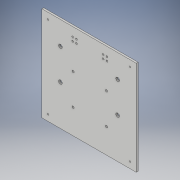
# Autodesk Inventor part: base_plate_v1
Saved by Autodesk Inventor 2019 (Build 230136000, 136)
## iProperties
Created: 2018-09-28
Part Number: base_plate_v1
Material: Generic
Document SubType Name: Modeling
Designer: Brian
Density: 1 g/cm^3
Appearance: Default
Author: Brian
Autodesk Inventor part; units mm, degrees
ref_plane "YZ Plane" through (0, 0, 0) normal (1, 0, 0) x (0, 1, 0)
ref_plane "XZ Plane" through (0, 0, 0) normal (0, 1, 0) x (-1, 0, 0)
ref_plane "XY Plane" through (0, 0, 0) normal (0, 0, 1) x (1, 0, 0)
sketch "Sketch1" plane through (0, 0, 0) normal (0, 0, 1) x (1, 0, 0)
  line L0 (0, 0) -> (304.8, 0)
  line L1 (304.8, 0) -> (304.8, 304.8)
  line L2 (304.8, 304.8) -> (0, 304.8)
  line L3 (0, 304.8) -> (0, 0)
  dimension "d0" = 304.8
  dimension "d1" = 304.8
  constraints: 8 end point, 2 parallel, 1 horizontal, 1 perpendicular
  measures "d0" distance of L2.end L1.end
  measures "d1" distance of L1.end L0.end
extrude "Extrusion1" add sketch "Sketch1" along normal blind 6
sketch "Sketch2" plane through (0, 0, 6) normal (0, 0, 1) x (1, 0, 0)
  line L0 (304.8, 0) -> (304.8, 304.8) projected
  line L1 (304.8, 304.8) -> (0, 304.8) projected
  point P0 (0, 0)
  point P1 (284.8, 284.8)
  dimension "d32" = 20
  dimension "d33" = 20
  measures "d32" distance from line of L0 point (284.8, 284.8)
  measures "d33" distance from line of L1 point (284.8, 284.8)
hole "Hole1" at (284.8, 284.8, 6) direction (0, 0, -1) diameter 5 end through all
sketch "Sketch3" plane through (0, 0, 6) normal (0, 0, 1) x (1, 0, 0)
  line L0 (0, 304.8) -> (0, 0) projected
  line L1 (304.8, 304.8) -> (0, 304.8) projected
  point P0 (20, 284.8)
  dimension "d34" = 20
  dimension "d35" = 20
  measures "d34" distance from line of L0 point (20, 284.8)
  measures "d35" distance from line of L1 point (20, 284.8)
hole "Hole2" at (20, 284.8, 6) direction (0, 0, -1) diameter 5 end through all
sketch "Sketch4" plane through (0, 0, 6) normal (0, 0, 1) x (1, 0, 0)
  line L0 (0, 0) -> (304.8, 0) projected
  line L1 (0, 304.8) -> (0, 0) projected
  point P0 (20, 20)
  dimension "d36" = 20
  dimension "d37" = 20
  measures "d36" distance from line of L0 point (20, 20)
  measures "d37" distance from line of L1 point (20, 20)
hole "Hole3" at (20, 20, 6) direction (0, 0, -1) diameter 5 end through all
sketch "Sketch5" plane through (0, 0, 6) normal (0, 0, 1) x (1, 0, 0)
  line L0 (0, 0) -> (304.8, 0) projected
  line L1 (304.8, 0) -> (304.8, 304.8) projected
  point P0 (284.8, 20)
  dimension "d38" = 20
  dimension "d39" = 20
  measures "d38" distance from line of L0 point (284.8, 20)
  measures "d39" distance from line of L1 point (284.8, 20)
hole "Hole4" at (284.8, 20, 6) direction (0, 0, -1) diameter 5 end through all
sketch "Sketch6" plane through (0, 0, 6) normal (0, 0, 1) x (1, 0, 0)
  line L0 (304.8, 304.8) -> (0, 304.8) projected
  line L1 (304.8, 0) -> (304.8, 304.8) projected
  point P0 (0, 0)
  point P1 (244.8, 229.8)
  dimension "d68" = 75
  dimension "d69" = 60
  measures "d68" distance from line of L0 point (244.8, 229.8)
  measures "d69" distance from line of L1 point (244.8, 229.8)
hole "Hole5" at (244.8, 229.8, 6) direction (0, 0, -1) diameter 12 end through all
sketch "Sketch7" plane through (0, 0, 6) normal (0, 0, 1) x (1, 0, 0)
  line L0 (304.8, 0) -> (304.8, 304.8) projected
  circle A0 centre (244.8, 229.8) radius 6 projected
  point P0 (0, 0)
  point P1 (244.8, 129.8)
  dimension "d72" = 60
  dimension "d73" = 100
  measures "d72" distance from line of L0 point (244.8, 129.8)
  measures "d73" distance of A0.centre point (244.8, 129.8)
hole "Hole6" at (244.8, 129.8, 6) direction (0, 0, -1) diameter 12 end through all
sketch "Sketch8" plane through (0, 0, 6) normal (0, 0, 1) x (1, 0, 0)
  line L0 (304.8, 304.8) -> (0, 304.8) projected
  line L1 (0, 304.8) -> (0, 0) projected
  point P0 (60, 229.8)
  dimension "d70" = 75
  dimension "d71" = 60
  measures "d70" distance from line of L0 point (60, 229.8)
  measures "d71" distance from line of L1 point (60, 229.8)
hole "Hole7" at (60, 229.8, 6) direction (0, 0, -1) diameter 12 end through all
sketch "Sketch9" plane through (0, 0, 6) normal (0, 0, 1) x (1, 0, 0)
  line L0 (0, 304.8) -> (0, 0) projected
  circle A0 centre (60, 229.8) radius 6 projected
  point P0 (60, 129.8)
  dimension "d74" = 60
  dimension "d75" = 100
  measures "d74" distance from line of L0 point (60, 129.8)
  measures "d75" distance of A0.centre point (60, 129.8)
hole "Hole8" at (60, 129.8, 6) direction (0, 0, -1) diameter 12 end through all
sketch "Sketch10" plane through (0, 0, 6) normal (0, 0, 1) x (1, 0, 0)
  line L0 (304.8, 304.8) -> (0, 304.8) projected
  line L1 (304.8, 0) -> (304.8, 304.8) projected
  line L2 (0, 304.8) -> (0, 0) projected
  point P0 (198.1, 275.8)
  point P1 (210.1, 275.8)
  point P2 (198.1, 263.8)
  point P3 (210.1, 263.8)
  point P4 (99.6, 275.8)
  point P5 (111.6, 275.8)
  point P6 (99.6, 263.8)
  point P7 (111.6, 263.8)
  dimension "d83" = 29
  dimension "d84" = 29
  dimension "d85" = 29
  dimension "d86" = 29
  dimension "d87" = 12
  dimension "d88" = 12
  dimension "d89" = 12
  dimension "d90" = 12
  dimension "d91" = 12
  dimension "d92" = 12
  dimension "d93" = 12
  dimension "d94" = 12
  dimension "d97" = 106.7
  dimension "d98" = 106.7
  dimension "d101" = 86.5
  dimension "d102" = 86.5
  measures "d83" distance from line of L0 point (210.1, 275.8)
  measures "d84" distance from line of L0 point (198.1, 275.8)
  measures "d85" distance from line of L0 point (111.6, 275.8)
  measures "d86" distance from line of L0 point (99.6, 275.8)
  measures "d87" distance of point (210.1, 275.8) point (210.1, 263.8)
  measures "d88" distance of point (198.1, 275.8) point (198.1, 263.8)
  measures "d89" distance of point (210.1, 263.8) point (198.1, 263.8)
  measures "d90" distance of point (210.1, 275.8) point (198.1, 275.8)
  measures "d91" distance of point (111.6, 275.8) point (99.6, 275.8)
  measures "d92" distance of point (111.6, 263.8) point (99.6, 263.8)
  measures "d93" distance of point (111.6, 275.8) point (111.6, 263.8)
  measures "d94" distance of point (99.6, 275.8) point (99.6, 263.8)
  measures "d97" distance from line of L1 point (198.1, 263.8)
  measures "d98" distance from line of L1 point (198.1, 275.8)
  measures "d101" distance of point (198.1, 275.8) point (111.6, 275.8)
  measures "d102" distance of point (198.1, 263.8) point (111.6, 263.8)
hole "Hole9" at (198.1, 275.8, 6) at (210.1, 275.8, 6) at (198.1, 263.8, 6) at (210.1, 263.8, 6) at (99.6, 275.8, 6) at (111.6, 275.8, 6) at (99.6, 263.8, 6) at (111.6, 263.8, 6) direction (0, 0, -1) diameter 3.1 end through all counterbore diameter 5.7 counterbore depth 3.5
sketch "Sketch11" plane through (0, 0, 6) normal (0, 0, 1) x (1, 0, 0)
  circle A0 centre (244.8, 229.8) radius 6 projected
  circle A1 centre (60, 229.8) radius 6 projected
  circle A2 centre (244.8, 129.8) radius 6 projected
  circle A3 centre (60, 129.8) radius 6 projected
  line L0 (304.8, 0) -> (304.8, 304.8) projected
  point P0 (0, 0)
  point P1 (208.8, 179.8)
  point P2 (208.8, 79.8)
  point P3 (100.8, 79.8)
  point P4 (100.8, 179.8)
  dimension "d110" = 108
  dimension "d111" = 108
  dimension "d112" = 50
  dimension "d113" = 50
  dimension "d116" = 96
  dimension "d117" = 96
  dimension "d118" = 100
  dimension "d119" = 100
  measures "d110" distance of point (208.8, 179.8) point (100.8, 179.8)
  measures "d111" distance of point (208.8, 79.8) point (100.8, 79.8)
  measures "d112" vertical distance of A0.centre point (208.8, 179.8)
  measures "d113" vertical distance of A1.centre point (100.8, 179.8)
  measures "d116" distance from line of L0 point (208.8, 79.8)
  measures "d117" distance from line of L0 point (208.8, 179.8)
  measures "d118" distance of point (208.8, 79.8) point (208.8, 179.8)
  measures "d119" distance of point (100.8, 79.8) point (100.8, 179.8)
hole "Hole10" at (208.8, 179.8, 6) at (208.8, 79.8, 6) at (100.8, 79.8, 6) at (100.8, 179.8, 6) direction (0, 0, -1) diameter 7 end through all
body "Solid1"
